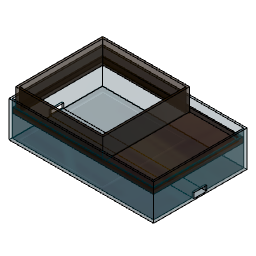
PumpkinAugen Arduino v2 (Autodesk Fusion 360 design; units mm, degrees)
Autodesk Fusion 360 part; units mm, degrees
sketch "Skizze1" plane through (0, 0, 0) normal (0, 1, 0) x (1, 0, 0)
  line L0 (27.5, -17.5) -> (-27.5, -17.5)
  line L1 (-27.5, -17.5) -> (-27.5, 17.5)
  line L2 (-27.5, 17.5) -> (27.5, 17.5)
  line L3 (27.5, 17.5) -> (27.5, -17.5)
  line L4 (27.5, -17.5) -> (-27.5, 17.5) construction
  line L5 (-27.5, -17.5) -> (27.5, 17.5) construction
  line L6 (6.3165, 16.3165) -> (-26.1835, 16.3165)
  line L7 (-26.1835, 16.3165) -> (-26.1835, -16.1835)
  line L8 (-26.1835, -16.1835) -> (6.3165, -16.1835)
  line L9 (6.3165, -16.1835) -> (6.3165, 16.3165)
  line L10 (6.3165, 16.3165) -> (-26.1835, -16.1835) construction
  line L11 (-26.1835, 16.3165) -> (6.3165, -16.1835) construction
  line L12 (7.0665, -16.9335) -> (-26.9335, -16.9335)
  line L13 (-26.9335, -16.9335) -> (-26.9335, 17.0665)
  line L14 (-26.9335, 17.0665) -> (7.0665, 17.0665)
  line L15 (7.0665, 17.0665) -> (7.0665, -16.9335)
  line L16 (7.0665, -16.9335) -> (-26.9335, 17.0665) construction
  line L17 (-26.9335, -16.9335) -> (7.0665, 17.0665) construction
  line L18 (27, -17) -> (-27, -17)
  line L19 (-27, -17) -> (-27, 17)
  line L20 (-27, 17) -> (27, 17)
  line L21 (27, 17) -> (27, -17)
  line L22 (27, -17) -> (-27, 17) construction
  line L23 (-27, -17) -> (27, 17) construction
  point P0 (-9.9335, 0.0665)
  point P1 (-9.9335, 0.0665)
  dimension "d1" = 55
  dimension "d2" = 35
  dimension "d3" = 32.5
  dimension "d4" = 32.5
  dimension "d5" = 1.3165
  dimension "d6" = 1.3165
  dimension "d7" = 34
  dimension "d8" = 34
  dimension "d9" = 34
  dimension "d10" = 54
  constraint perpendicular L0 L1
  constraint parallel L0 L2
  constraint parallel L1 L3
  constraint horizontal L0
  constraint coincident L4 origin
  constraint coincident L5 origin
  constraint perpendicular L6 L7
  constraint parallel L6 L8
  constraint parallel L7 L9
  constraint horizontal L6
  constraint coincident L10 P1
  constraint coincident L11 P1
  constraint perpendicular L12 L13
  constraint parallel L12 L14
  constraint parallel L13 L15
  constraint horizontal L12
  constraint coincident L16 P1
  constraint coincident L17 P1
  constraint coincident P1 P0
  constraint perpendicular L18 L19
  constraint parallel L18 L20
  constraint parallel L19 L21
  constraint horizontal L18
  constraint coincident L22 origin
  constraint coincident L23 origin
  measures "d1" distance of L1.end L2.end
  measures "d2" distance of L0.end L1.end
  measures "d3" distance of L7.end L8.end
  measures "d4" distance of L6.end L7.end
  measures "d5" vertical distance of L0.end L7.end
  measures "d6" horizontal distance of L1.end L6.end
  measures "d7" distance of L13.end L14.end
  measures "d8" distance of L12.start L14.end
  measures "d9" distance of L18.start L20.end
  measures "d10" distance of L18.start L18.end
extrude "Extrusion1" add sketch "Skizze1" along normal blind 0.5 contours L12 L13 L15 L18 L19 L20 L21 makes body 1
extrude "Extrusion2" add sketch "Skizze1" along normal blind 9 contours L12 L13 L15 L20 bodies 1
extrude "Extrusion3" add sketch "Skizze1" along normal blind 2 separate body contours L0 L1 L2 L3 makes body 2
sketch "Skizze2" plane through (0, 0, 0) normal (0, 1, 0) x (1, 0, 0)
  line L0 (27.6, -17.6) -> (-27.6, -17.6)
  line L1 (-27.6, -17.6) -> (-27.6, 17.6)
  line L2 (-27.6, 17.6) -> (27.6, 17.6)
  line L3 (27.6, 17.6) -> (27.6, -17.6)
  line L4 (27.6, -17.6) -> (-27.6, 17.6) construction
  line L5 (-27.6, -17.6) -> (27.6, 17.6) construction
  line L6 (28.25, -18.25) -> (-28.25, -18.25)
  line L7 (-28.25, -18.25) -> (-28.25, 18.25)
  line L8 (-28.25, 18.25) -> (28.25, 18.25)
  line L9 (28.25, 18.25) -> (28.25, -18.25)
  line L10 (28.25, -18.25) -> (-28.25, 18.25) construction
  line L11 (-28.25, -18.25) -> (28.25, 18.25) construction
  dimension "d17" = 35.2
  dimension "d18" = 55.2
  dimension "d19" = 56.5
  dimension "d20" = 36.5
  constraint perpendicular L0 L1
  constraint parallel L0 L2
  constraint parallel L1 L3
  constraint horizontal L0
  constraint coincident L4 origin
  constraint coincident L5 origin
  constraint perpendicular L6 L7
  constraint parallel L6 L8
  constraint parallel L7 L9
  constraint horizontal L6
  constraint coincident L10 origin
  constraint coincident L11 origin
  measures "d17" distance of L0.end L1.end
  measures "d18" distance of L1.end L2.end
  measures "d19" distance of L7.end L8.end
  measures "d20" distance of L6.end L7.end
extrude "Extrusion4" add sketch "Skizze2" along normal blind 0.5 separate body contours L0 L1 L2 L3 makes body 3
extrude "Extrusion5" add sketch "Skizze2" along normal blind 14 bodies 3
sketch "Skizze3" plane through (28.25, 0, 0) normal (1, 0, 0) x (0, 0, -1)
  line L0 (-18.25, 0) -> (18.25, 0)
  line L1 (18.25, 0) -> (18.25, 14)
  line L2 (18.25, 14) -> (-18.25, 14)
  line L3 (-18.25, 14) -> (-18.25, 0)
  line L4 (2.5, 0.4582) -> (-2.5, 0.4582)
  line L5 (-2.5, 0.4582) -> (-2.5, 2.4582)
  line L6 (-2.5, 2.4582) -> (2.5, 2.4582)
  line L7 (2.5, 2.4582) -> (2.5, 0.4582)
  line L8 (2.5, 0.4582) -> (-2.5, 2.4582) construction
  line L9 (-2.5, 0.4582) -> (2.5, 2.4582) construction
  point P0 (0, 1.4582)
  dimension "d25" = 5
  dimension "d26" = 2
  constraint perpendicular L4 L5
  constraint parallel L4 L6
  constraint parallel L5 L7
  constraint horizontal L4
  constraint coincident L8 P0
  constraint coincident L9 P0
  measures "d25" distance of L5.end L6.end
  measures "d26" distance of L4.end L5.end
extrude "Extrusion6" cut sketch "Skizze3" against normal blind 70 contours L4 L5 L6 L7 bodies 3
combine "Kombinieren1" operation add target body 1 tool bodies 2
move_body "Verschieben1" bodies 1 to x (1, 0, 0) y (0, 1, 0) z (0, 0, 1) at (0, 9, 0)
sketch "Skizze4" plane through (0, 9, 0) normal (0, -1, 0) x (1, 0, 0)
  line L0 (-27.5, -17.5) -> (27.5, -17.5)
  line L1 (27.5, -17.5) -> (27.5, 17.5)
  line L2 (27.5, 17.5) -> (-27.5, 17.5)
  line L3 (-27.5, 17.5) -> (-27.5, -17.5)
  line L4 (6.3165, 16.1835) -> (6.3165, -16.3165)
  line L5 (6.3165, -16.3165) -> (-26.1835, -16.3165)
  line L6 (-26.1835, -16.3165) -> (-26.1835, 16.1835)
  line L7 (-26.1835, 16.1835) -> (6.3165, 16.1835)
  line L8 (-26.9335, -17) -> (7.0665, -17)
  line L9 (7.0665, -17) -> (7.0665, -17.0665)
  line L10 (7.0665, -17.0665) -> (-26.9335, -17.0665)
  line L11 (-26.9335, -17.0665) -> (-26.9335, -17)
  line L12 (21.4325, -16.5665) -> (6.4325, -16.5665)
  line L13 (6.4325, -16.5665) -> (6.4325, 16.4335)
  line L14 (6.4325, 16.4335) -> (21.4325, 16.4335)
  line L15 (21.4325, 16.4335) -> (21.4325, -16.5665)
  line L16 (21.4325, -16.5665) -> (6.4325, 16.4335) construction
  line L17 (6.4325, -16.5665) -> (21.4325, 16.4335) construction
  point P0 (13.9325, -0.0665)
  dimension "d29" = 33
  dimension "d30" = 15
  constraint perpendicular L12 L13
  constraint parallel L12 L14
  constraint parallel L13 L15
  constraint horizontal L12
  constraint coincident L16 P0
  constraint coincident L17 P0
  measures "d29" distance of L12.end L13.end
  measures "d30" distance of L13.end L14.end
equation "d6 = d5"
equation "d7 = d4 + 1.5 mm"
equation "d8 = d7"
equation "d9 = d2 - 1 mm"
equation "d10 = d1 - 1 mm"
